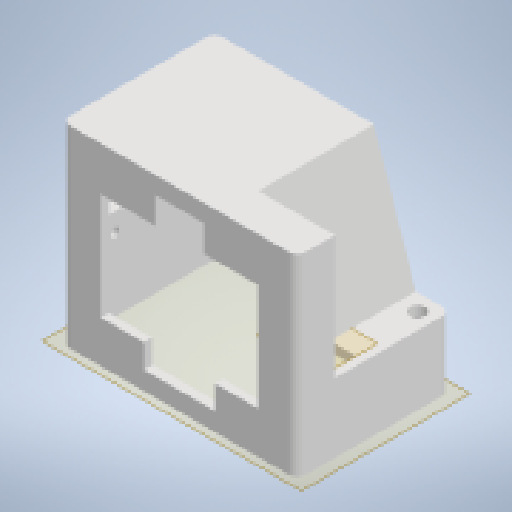
# Autodesk Inventor part: Gehaeuse_oben
Saved by Autodesk Inventor 2024 (Build 280153000, 153)
## iProperties
Created: 2025-04-09
Part Number: Gehaeuse_oben
Material: Generisch
Document SubType Name: Modeling
Designer: erikt
Density: 1 g/cm^3
Appearance: Vorgabe
Author: erikt
Autodesk Inventor part; units mm, degrees
ref_plane "YZ Plane" through (0, 0, 0) normal (1, 0, 0) x (0, 1, 0)
ref_plane "XZ Plane" through (0, 0, 0) normal (0, 1, 0) x (-1, 0, 0)
ref_plane "XY Plane" through (0, 0, 0) normal (0, 0, 1) x (1, 0, 0)
ref_plane "Arbeitsebene1" through (0, 0, 0) normal (0, 0, 1) x (1, 0, 0)
sketch "Skizze1" plane through (0, 0, 0) normal (0, 0, 1) x (1, 0, 0)
  arc A0 (-23.82, 16.765) -> (-25.82, 14.765) centre (-23.82, 14.765) ccw projected
  line L0 (-25.82, -14.765) -> (-25.82, 14.765) projected
  arc A1 (-25.82, -14.765) -> (-23.82, -16.765) centre (-23.82, -14.765) ccw projected
  line L1 (23.82, -16.765) -> (-23.82, -16.765) projected
  arc A2 (23.82, -16.765) -> (25.82, -14.765) centre (23.82, -14.765) ccw projected
  line L2 (25.82, 14.765) -> (25.82, -14.765) projected
  arc A3 (25.82, 14.765) -> (23.82, 16.765) centre (23.82, 14.765) ccw projected
  line L3 (-23.82, 16.765) -> (23.82, 16.765) projected
  arc A4 (23.82, -15.765) -> (24.82, -14.765) centre (23.82, -14.765) ccw projected
  line L4 (-23.82, -15.765) -> (23.82, -15.765) projected
  arc A5 (-24.82, -14.765) -> (-23.82, -15.765) centre (-23.82, -14.765) ccw projected
  line L5 (-24.82, 14.765) -> (-24.82, -14.765) projected
  arc A6 (-23.82, 15.765) -> (-24.82, 14.765) centre (-23.82, 14.765) ccw projected
  line L6 (23.82, 15.765) -> (-23.82, 15.765) projected
  arc A7 (24.82, 14.765) -> (23.82, 15.765) centre (23.82, 14.765) ccw projected
  line L7 (24.82, -14.765) -> (24.82, 14.765) projected
  arc A8 (-23.82, 15.965) -> (-25.02, 14.765) centre (-23.82, 14.765) ccw
  line L8 (-25.02, 14.765) -> (-25.02, -14.765)
  arc A9 (-25.02, -14.765) -> (-23.82, -15.965) centre (-23.82, -14.765) ccw
  line L9 (-23.82, -15.965) -> (23.82, -15.965)
  arc A10 (23.82, -15.965) -> (25.02, -14.765) centre (23.82, -14.765) ccw
  line L10 (25.02, -14.765) -> (25.02, 14.765)
  arc A11 (25.02, 14.765) -> (23.82, 15.965) centre (23.82, 14.765) ccw
  line L11 (23.82, 15.965) -> (-23.82, 15.965)
  point P0 (0, 0)
  dimension "d0" = 0.2
  constraints: 8 end point, 8 point on circle, 4 centre point, 7 other
  measures "d0" distance between parallel lines of L6 L11
extrude "Extrusion1" add sketch "Skizze1" along normal blind 2.2 contours L3 A3 L2 A2 L1 A1 L0 A0
sketch "Skizze2" plane through (0, 0, 2.2) normal (0, 0, 1) x (1, 0, 0)
  line L0 (23.82, 16.765) -> (-23.82, 16.765) projected
  line L1 (23.82, 14.765) -> (-23.82, 14.765) projected
  arc A0 (-24.82, -14.765) -> (-23.82, -15.765) centre (-23.82, -14.765) ccw projected
  line L2 (-23.82, -15.765) -> (23.82, -15.765) projected
  arc A1 (23.82, -15.765) -> (24.82, -14.765) centre (23.82, -14.765) ccw projected
  line L3 (24.82, -14.765) -> (24.82, 14.765) projected
  arc A2 (24.82, 14.765) -> (23.82, 15.765) centre (23.82, 14.765) ccw projected
  line L4 (23.82, 15.765) -> (-23.82, 15.765) projected
  arc A3 (-23.82, 15.765) -> (-24.82, 14.765) centre (-23.82, 14.765) ccw projected
  line L5 (-24.82, 14.765) -> (-24.82, -14.765) projected
  line L6 (-23.82, 14.765) -> (-23.82, -14.765) projected
  line L7 (23.82, 14.765) -> (-23.82, 14.765) projected
  line L8 (23.82, -14.765) -> (23.82, 14.765) projected
  line L9 (-23.82, -14.765) -> (23.82, -14.765) projected
  line L10 (23.82, 16.765) -> (-23.82, 16.765) projected
  arc A4 (-23.82, 16.765) -> (-25.82, 14.765) centre (-23.82, 14.765) ccw projected
  line L11 (-25.82, 14.765) -> (-25.82, -14.765) projected
  arc A5 (-25.82, -14.765) -> (-23.82, -16.765) centre (-23.82, -14.765) ccw projected
  line L12 (-23.82, -16.765) -> (23.82, -16.765) projected
  arc A6 (23.82, -16.765) -> (25.82, -14.765) centre (23.82, -14.765) ccw projected
  line L13 (25.82, -14.765) -> (25.82, 14.765) projected
  arc A7 (25.82, 14.765) -> (23.82, 16.765) centre (23.82, 14.765) ccw projected
  line L14 (-23.82, 15.965) -> (23.82, 15.965) projected
  arc A8 (25.02, 14.765) -> (23.82, 15.965) centre (23.82, 14.765) ccw projected
  line L15 (25.02, 14.765) -> (25.02, -14.765) projected
  arc A9 (23.82, -15.965) -> (25.02, -14.765) centre (23.82, -14.765) ccw projected
  line L16 (23.82, -15.965) -> (-23.82, -15.965) projected
  arc A10 (-25.02, -14.765) -> (-23.82, -15.965) centre (-23.82, -14.765) ccw projected
  line L17 (-25.02, -14.765) -> (-25.02, 14.765) projected
  arc A11 (-23.82, 15.965) -> (-25.02, 14.765) centre (-23.82, 14.765) ccw projected
  point P0 (0, 0)
extrude "Extrusion2" add sketch "Skizze2" along normal blind 38 contours A7 L13 A6 L12 A5 L11 A4 L0 | L5 A3 L4 A2 L3 A1 L2 A0 | L14 A8 L15 A9 L16 A10 L17 A11
sketch "Skizze3" plane through (-23.82, -16.765, 0) normal (0, -1, 0) x (1, 0, 0)
  line L0 (-2, 0) -> (-2, 40.2) projected
  line L1 (0, 40.2) -> (-2, 40.2) projected
  line L2 (0, 40.2) -> (47.64, 40.2) projected
  line L3 (49.64, 0) -> (49.64, 40.2) projected
  line L4 (49.64, 40.2) -> (47.64, 40.2) projected
  line L5 (49.64, 0) -> (47.64, 0) projected
  line L6 (0, 0) -> (47.64, 0) projected
  line L7 (-2, 0) -> (0, 0) projected
  line L8 (5.82, 38.2) -> (41.82, 38.2)
  line L9 (41.82, 38.2) -> (41.82, 4.2)
  line L10 (41.82, 4.2) -> (5.82, 4.2)
  line L11 (5.82, 4.2) -> (5.82, 38.2)
  point P0 (23.82, 0)
  dimension "d5" = 36
  dimension "d6" = 34
  dimension "d7" = 2
  dimension "d8" = 7.82
  dimension "d9" = 7.82
  constraints: 8 end point, 2 parallel, 1 horizontal, 1 perpendicular
  measures "d5" distance of L9.end L10.end
  measures "d6" distance of L8.end L9.end
  measures "d7" distance between parallel lines of L2 L8
  measures "d8" distance between parallel lines of L11 L0
  measures "d9" distance between parallel lines of L3 L9
extrude "Extrusion3" cut sketch "Skizze3" against normal up to surface (2 mm away) contours L8 L9 L10 L11
sketch "Skizze4" plane through (-23.82, -16.765, 0) normal (0, -1, 0) x (1, 0, 0)
  line L0 (5.82, 4.2) -> (5.82, 38.2) projected
  line L1 (5.82, 4.2) -> (5.82, 38.2) projected
  line L2 (5.82, 38.2) -> (41.82, 38.2) projected
  line L3 (41.82, 38.2) -> (41.82, 4.2) projected
  line L4 (41.82, 4.2) -> (5.82, 4.2) projected
  line L5 (0, 0) -> (47.64, 0) projected
  line L6 (47.64, 0) -> (47.64, 40.2) projected
  line L7 (0, 40.2) -> (47.64, 40.2) projected
  line L8 (0, 0) -> (0, 40.2) projected
  line L9 (42.02, 38.4) -> (5.62, 38.4)
  line L10 (5.62, 38.4) -> (5.62, 4)
  line L11 (5.62, 4) -> (42.02, 4)
  line L12 (42.02, 4) -> (42.02, 38.4)
  point P0 (23.82, 0)
  dimension "d12" = 0.2
  constraints: 8 end point, 3 other
  measures "d12" distance between parallel lines of L2 L9
extrude "Extrusion4" cut sketch "Skizze4" against normal up to surface (2 mm away) contours L12 L11 L10 L9
sketch "Skizze5" plane through (-23.82, -16.765, 0) normal (0, -1, 0) x (1, 0, 0)
  line L0 (5.62, 38.4) -> (42.02, 38.4) projected
  line L1 (42.02, 38.4) -> (42.02, 4) projected
  line L2 (42.02, 4) -> (5.62, 4) projected
  line L3 (5.62, 4) -> (5.62, 38.4) projected
  line L4 (0, 0) -> (47.64, 0) projected
  line L5 (47.64, 0) -> (47.64, 40.2) projected
  line L6 (0, 40.2) -> (47.64, 40.2) projected
  line L7 (0, 0) -> (0, 40.2) projected
  line L8 (31.32, 4.2) -> (31.32, 9.2) projected
  line L9 (31.32, 4.2) -> (41.82, 4.2) projected
  line L10 (41.82, 4.2) -> (41.82, 38.2) projected
  line L11 (41.82, 38.2) -> (5.82, 38.2) projected
  line L12 (5.82, 38.2) -> (5.82, 4.2) projected
  line L13 (5.82, 4.2) -> (16.32, 4.2) projected
  line L14 (16.32, 9.2) -> (16.32, 4.2) projected
  line L15 (31.32, 9.2) -> (16.32, 9.2) projected
  line L16 (40.82, 32.4) -> (6.82, 32.4) projected
  line L17 (40.82, 9.4) -> (40.82, 32.4) projected
  line L18 (6.82, 9.4) -> (40.82, 9.4) projected
  line L19 (6.82, 32.4) -> (6.82, 9.4) projected
  circle A0 centre (39.2325, 35.4875) radius 2.0875 projected
  circle A1 centre (8.4075, 35.4875) radius 2.0875 projected
  circle A2 centre (8.4075, 6.9125) radius 2.0875 projected
  circle A3 centre (39.2325, 6.9125) radius 2.0875 projected
  line L20 (28.63, 35.95) -> (26.63, 35.95) projected
  line L21 (26.63, 35.95) -> (26.63, 37.95) projected
  line L22 (26.63, 37.95) -> (28.63, 37.95) projected
  line L23 (28.63, 37.95) -> (28.63, 35.95) projected
  line L24 (26.09, 35.95) -> (24.09, 35.95) projected
  line L25 (24.09, 35.95) -> (24.09, 37.95) projected
  line L26 (24.09, 37.95) -> (26.09, 37.95) projected
  line L27 (26.09, 37.95) -> (26.09, 35.95) projected
  line L28 (21.55, 35.95) -> (21.55, 37.95) projected
  line L29 (21.55, 37.95) -> (23.55, 37.95) projected
  line L30 (23.55, 37.95) -> (23.55, 35.95) projected
  line L31 (23.55, 35.95) -> (21.55, 35.95) projected
  line L32 (19.01, 37.95) -> (21.01, 37.95) projected
  line L33 (21.01, 37.95) -> (21.01, 35.95) projected
  line L34 (21.01, 35.95) -> (19.01, 35.95) projected
  line L35 (19.01, 35.95) -> (19.01, 37.95) projected
  line L36 (6.62, 32.6) -> (41.02, 32.6)
  line L37 (41.02, 32.6) -> (41.02, 9.2)
  line L38 (41.02, 9.2) -> (6.62, 9.2)
  line L39 (6.62, 9.2) -> (6.62, 32.6)
  line L40 (19.01, 35.95) -> (28.63, 35.95)
  line L41 (28.63, 35.95) -> (28.63, 37.95)
  line L42 (28.63, 37.95) -> (19.01, 37.95)
  line L43 (19.01, 37.95) -> (19.01, 35.95)
  line L44 (29.13, 35.45) -> (18.51, 35.45)
  line L45 (18.51, 35.45) -> (18.51, 38.45)
  line L46 (18.51, 38.45) -> (29.13, 38.45)
  line L47 (29.13, 38.45) -> (29.13, 35.45)
  line L48 (16.02, 4.5) -> (6.12, 4.5)
  line L49 (6.12, 4.5) -> (6.12, 37.9)
  line L50 (6.12, 37.9) -> (41.52, 37.9)
  line L51 (41.52, 37.9) -> (41.52, 4.5)
  line L52 (41.52, 4.5) -> (31.62, 4.5)
  line L53 (31.62, 4.5) -> (31.62, 9.5)
  line L54 (31.62, 9.5) -> (16.02, 9.5)
  line L55 (16.02, 9.5) -> (16.02, 4.5)
  line L56 (16.02, 4.5) -> (16.02, 4)
  line L57 (31.62, 4.5) -> (31.62, 4)
  point P0 (23.82, 0)
  point P1 (31.62, 9.2)
  point P2 (29.13, 38.4)
  point P3 (18.51, 38.4)
  point P4 (16.02, 9.2)
  dimension "d15" = 0.2
  dimension "d16" = 0.5
  dimension "d17" = 0.3
  constraints: 44 end point, 4 parallel, 4 perpendicular, 2 point on line, 1 horizontal, 13 other
  measures "d15" distance between parallel lines of L16 L36
  measures "d16" distance between parallel lines of L40 L44
  measures "d17" distance between parallel lines of L14 L55
extrude "Extrusion5" add sketch "Skizze5" against normal blind 1.8 contours L0 L45 L11 L12 L13 L56 L2 L3 | L0 L1 L2 L57 L9 L10 L11 L47 | L45 L50 L49 L48 L56 L13 L12 L11 | L11 L10 L9 L57 L52 L51 L50 L47 | L45 L44 L47 L50 L51 L52 L53 L38 L37 L36 L39 L55 L48 L49 | A0 | A1 | A2 | A3
sketch "Skizze6" plane through (-23.82, 16.765, 0) normal (0, 1, 0) x (1, 0, 0)
  arc A0 (21.6432, -14.6) -> (20.1432, -13.1) centre (20.1432, -14.6) ccw projected
  line L0 (21.6432, -14.8) -> (21.6432, -14.6) projected
  arc A1 (20.1432, -16.3) -> (21.6432, -14.8) centre (20.1432, -14.8) ccw projected
  line L1 (14.1432, -16.3) -> (20.1432, -16.3) projected
  arc A2 (12.6432, -14.8) -> (14.1432, -16.3) centre (14.1432, -14.8) ccw projected
  line L2 (12.6432, -14.8) -> (12.6432, -14.6) projected
  arc A3 (14.1432, -13.1) -> (12.6432, -14.6) centre (14.1432, -14.6) ccw projected
  line L3 (20.1432, -13.1) -> (14.1432, -13.1) projected
  arc A4 (14.1432, -11.5) -> (11.0432, -14.6) centre (14.1432, -14.6) ccw
  line L4 (11.0432, -14.6) -> (11.0432, -14.8)
  arc A5 (11.0432, -14.8) -> (14.1432, -17.9) centre (14.1432, -14.8) ccw
  line L5 (14.1432, -17.9) -> (20.1432, -17.9)
  arc A6 (20.1432, -17.9) -> (23.2432, -14.8) centre (20.1432, -14.8) ccw
  line L6 (23.2432, -14.8) -> (23.2432, -14.6)
  arc A7 (23.2432, -14.6) -> (20.1432, -11.5) centre (20.1432, -14.6) ccw
  line L7 (20.1432, -11.5) -> (14.1432, -11.5)
  point P0 (23.82, 0)
  dimension "d20" = 1.6
  constraints: 8 end point, 8 point on circle, 4 centre point, 7 other
  measures "d20" distance between parallel lines of L3 L7
extrude "Extrusion6" cut sketch "Skizze6" against normal up to surface (2 mm away) contours L0 A1 L1 A2 L2 A3 L3 A0 | L7 A7 L6 A6 L5 A5 L4 A4
sketch "Skizze7" plane through (-23.82, -16.765, 0) normal (0, -1, 0) x (1, 0, 0)
  line L0 (31.62, 4) -> (16.02, 4) projected
  line L1 (16.02, 4) -> (16.02, 9.2) projected
  line L2 (16.02, 9.2) -> (6.62, 9.2) projected
  line L3 (6.62, 9.2) -> (6.62, 32.6) projected
  line L4 (6.62, 32.6) -> (41.02, 32.6) projected
  line L5 (41.02, 32.6) -> (41.02, 9.2) projected
  line L6 (41.02, 9.2) -> (31.62, 9.2) projected
  line L7 (31.62, 9.2) -> (31.62, 4) projected
  line L8 (29.13, 38.4) -> (29.13, 35.45) projected
  line L9 (29.13, 35.45) -> (18.51, 35.45) projected
  line L10 (18.51, 35.45) -> (18.51, 38.4) projected
  line L11 (18.51, 38.4) -> (29.13, 38.4) projected
  line L12 (0, 0) -> (47.64, 0) projected
  line L13 (47.64, 0) -> (47.64, 40.2) projected
  line L14 (0, 40.2) -> (47.64, 40.2) projected
  line L15 (0, 0) -> (0, 40.2) projected
  line L16 (18.51, 35.45) -> (29.13, 35.45)
  line L17 (29.13, 35.45) -> (29.13, 32.6)
  line L18 (29.13, 32.6) -> (18.51, 32.6)
  line L19 (18.51, 32.6) -> (18.51, 35.45)
  point P0 (23.82, 0)
  constraints: 8 end point, 2 parallel, 1 horizontal, 1 perpendicular, 1 point on line
extrude "Extrusion7" cut sketch "Skizze7" against normal up to surface (2 mm away) contours L4 L19 L9 L17
sketch "Skizze8" plane through (-23.82, -14.765, 2.2) normal (0, 1, 0) x (1, 0, 0)
  line L0 (41.82, -2) -> (41.82, -36) projected
  line L1 (41.82, -19) -> (47.64, -19)
  line L2 (47.64, 0) -> (47.64, -38) projected
  line L3 (45.98, -23) -> (43.48, -23)
  line L4 (43.48, -23) -> (43.48, -15)
  line L5 (43.48, -15) -> (45.98, -15)
  line L6 (45.98, -15) -> (45.98, -23)
  line L7 (45.98, -23) -> (43.48, -15) construction
  line L8 (43.48, -23) -> (45.98, -15) construction
  line L9 (5.82, -36) -> (5.82, -2) projected
  line L10 (5.62, -36.2) -> (5.62, -1.8) projected
  line L11 (5.62, -19) -> (0, -19)
  line L12 (0, 2.2) -> (0, -38) projected
  line L13 (4.06, -23) -> (1.56, -23)
  line L14 (1.56, -23) -> (1.56, -15)
  line L15 (1.56, -15) -> (4.06, -15)
  line L16 (4.06, -15) -> (4.06, -23)
  line L17 (4.06, -23) -> (1.56, -15) construction
  line L18 (1.56, -23) -> (4.06, -15) construction
  point P0 (23.82, 2.2)
  point P1 (44.73, -19)
  point P2 (2.81, -19)
  dimension "d25" = 2.5
  dimension "d26" = 8
  dimension "d27" = 2.5
  dimension "d28" = 8
  constraints: 28 end point, 9 midpoint, 4 parallel, 3 horizontal, 2 perpendicular, 1 point on line
  measures "d25" distance of L4.end L5.end
  measures "d26" distance of L3.end L4.end
  measures "d27" distance of L14.end L15.end
  measures "d28" distance of L13.end L14.end
extrude "Extrusion8" add sketch "Skizze8" along normal blind 5.5
sketch "Skizze9" plane through (19.66, -14.765, 17.2) normal (-1, 0, 0) x (0, 0, 1)
  line L0 (8, 0) -> (0, 0) projected
  line L1 (8, 0) -> (8, 5.5) projected
  line L2 (0, 5.5) -> (8, 5.5) projected
  line L3 (0, 0) -> (0, 5.5) projected
  line L4 (0, 0) -> (8, 0) projected
  line L5 (0, 0) -> (0, 5.5) projected
  line L6 (8, 5.5) -> (0, 5.5) projected
  line L7 (8, 0) -> (8, 5.5) projected
  line L8 (8, 5.5) -> (0, 5.5)
  line L9 (0, 5.5) -> (0, 2)
  line L10 (0, 2) -> (8, 2)
  line L11 (8, 2) -> (8, 5.5)
  line L12 (8, 2) -> (0, 5.5)
  line L13 (0, 5.5) -> (8, 5.5) projected
  line L14 (0, 2) -> (8, 5.5)
  circle A0 centre (4, 3.75) radius 1
  point P0 (-17.2, 14.765)
  dimension "d31" = 3.5
  dimension "d32" = 2
  constraints: 12 end point, 2 parallel, 1 centre point, 1 horizontal, 1 midpoint, 1 perpendicular, 1 point on line
  measures "d31" distance of L9.end L8.end
  measures "d32" diameter of A0
extrude "Extrusion9" cut sketch "Skizze9" against normal up to surface (2.5 mm away) contours A0 L14 L12 | L12 L14 A0 | A0 L12 L14 | L14 L12 A0
sketch "Skizze10" plane through (-19.76, -14.765, 25.2) normal (1, 0, 0) x (0, 0, -1)
  circle A0 centre (4, 3.75) radius 1 projected
  point P0 (25.2, 14.765)
extrude "Extrusion10" cut sketch "Skizze10" against normal up to surface (2.5 mm away)
sketch "Skizze11" plane through (-23.82, -9.265, 2.2) normal (0, 1, 0) x (1, 0, 0)
  line L0 (45.98, -23) -> (45.98, -15) projected
  line L1 (45.98, -15) -> (43.48, -15) projected
  line L2 (43.48, -15) -> (43.48, -23) projected
  line L3 (43.48, -23) -> (45.98, -23) projected
  line L4 (1.56, -15) -> (1.56, -23) projected
  line L5 (1.56, -23) -> (4.06, -23) projected
  line L6 (4.06, -23) -> (4.06, -15) projected
  line L7 (4.06, -15) -> (1.56, -15) projected
  point P0 (23.82, 2.2)
extrude "Extrusion11" add sketch "Skizze11" along normal blind 1
fillet "Rundung1" radius 2 4 edges at (-21.01, -8.265, 25.2) (20.91, -8.265, 25.2) (-21.01, -8.265, 17.2) (20.91, -8.265, 17.2)
ref_plane "Arbeitsebene2" through (9.72, -3.175, 15.1205) normal (0, 0, 1) x (0, -1, 0)
sketch "Skizze12" plane through (9.72, -3.175, 15.1205) normal (0, 0, 1) x (0, -1, 0)
  line L0 (5.35, 0) -> (5.35, 13.5) projected
  line L1 (11.59, 16.1) -> (-17.94, 16.1) projected
  line L2 (-17.94, 14.1) -> (11.59, 14.1) projected
  line L3 (5.35, 0) -> (-19.94, 0)
  line L4 (-19.94, 0) -> (-19.94, 16.1)
  line L5 (-19.94, 16.1) -> (5.35, 16.1)
  line L6 (5.35, 16.1) -> (5.35, 0)
  point P0 (-3.175, -9.72)
  point P1 (5.35, 16.1)
  point P2 (-17.94, 16.1)
  constraints: 8 end point, 2 parallel, 1 horizontal, 1 perpendicular
extrude "Extrusion12" cut sketch "Skizze12" along normal up to surface (25.0795 mm away)
sketch "Skizze13" plane through (-23.82, 16.765, 0) normal (0, 1, 0) x (1, 0, 0)
  line L0 (33.54, -15.1205) -> (47.64, -15.1205) projected
  line L1 (47.64, 0) -> (47.64, -15.1205) projected
  line L2 (47.64, 0) -> (0, 0) projected
  line L3 (0, 0) -> (0, -40.2) projected
  line L4 (33.54, -40.2) -> (0, -40.2) projected
  line L5 (33.54, -40.2) -> (33.54, -15.1205) projected
  arc A0 (23.2432, -14.6) -> (20.1432, -11.5) centre (20.1432, -14.6) ccw projected
  line L6 (23.2432, -14.6) -> (23.2432, -14.8) projected
  arc A1 (20.1432, -17.9) -> (23.2432, -14.8) centre (20.1432, -14.8) ccw projected
  line L7 (20.1432, -17.9) -> (14.1432, -17.9) projected
  arc A2 (11.0432, -14.8) -> (14.1432, -17.9) centre (14.1432, -14.8) ccw projected
  line L8 (11.0432, -14.8) -> (11.0432, -14.6) projected
  arc A3 (14.1432, -11.5) -> (11.0432, -14.6) centre (14.1432, -14.6) ccw projected
  line L9 (14.1432, -11.5) -> (20.1432, -11.5) projected
  line L10 (47.64, -15.1205) -> (49.64, -15.1205) projected
  line L11 (49.64, 0) -> (49.64, -15.1205) projected
  line L12 (49.64, 0) -> (47.64, 0) projected
  line L13 (47.64, 0) -> (47.64, -15.1205) projected
  line L14 (47.64, -40.2) -> (47.64, -15.1205) projected
  line L15 (49.64, -40.2) -> (47.64, -40.2) projected
  line L16 (49.64, -15.1205) -> (49.64, -40.2) projected
  line L17 (47.64, -15.1205) -> (49.64, -15.1205) projected
  line L18 (1.56, -17.2) -> (4.06, -17.2) projected
  line L19 (4.06, -17.2) -> (4.06, -25.2) projected
  line L20 (4.06, -25.2) -> (1.56, -25.2) projected
  line L21 (1.56, -25.2) -> (1.56, -17.2) projected
  line L22 (45.98, -25.2) -> (43.48, -25.2) projected
  line L23 (43.48, -25.2) -> (43.48, -17.2) projected
  line L24 (43.48, -17.2) -> (45.98, -17.2) projected
  line L25 (45.98, -17.2) -> (45.98, -25.2) projected
  line L26 (42.02, -38.4) -> (5.62, -38.4) projected
  line L27 (5.62, -38.4) -> (5.62, -4) projected
  line L28 (5.62, -4) -> (42.02, -4) projected
  line L29 (42.02, -4) -> (42.02, -38.4) projected
  line L30 (47.64, -2.2) -> (0, -2.2) projected
  line L31 (0, -2.2) -> (0, -40.2) projected
  line L32 (47.64, -40.2) -> (0, -40.2) projected
  line L33 (47.64, -2.2) -> (47.64, -40.2) projected
  line L34 (43.435, -12.1206) -> (42.94, -12.1206) projected
  line L35 (42.02, -15.1205) -> (33.54, -40.2)
  point P0 (23.82, 0)
  constraints: 2 end point, 2 point on line
extrude "Extrusion13" add sketch "Skizze13" against normal up to surface (2 mm away) contours L0 L35 L26 L5 | L26 L35 L5
sketch "Skizze15" plane through (0, 0, 40.2) normal (0, 0, 1) x (1, 0, 0)
  line L0 (25.82, -8.525) -> (23.82, -8.525) projected
  line L1 (23.82, -8.525) -> (23.82, -14.765) projected
  line L2 (23.82, -14.765) -> (-23.82, -14.765) projected
  line L3 (-23.82, -14.765) -> (-23.82, 14.765) projected
  line L4 (-23.82, 14.765) -> (9.72, 14.765) projected
  line L5 (9.72, 14.765) -> (9.72, 16.765) projected
  line L6 (9.72, 16.765) -> (-23.82, 16.765) projected
  arc A0 (-23.82, 16.765) -> (-25.82, 14.765) centre (-23.82, 14.765) ccw projected
  line L7 (-25.82, 14.765) -> (-25.82, -14.765) projected
  arc A1 (-25.82, -14.765) -> (-23.82, -16.765) centre (-23.82, -14.765) ccw projected
  line L8 (-23.82, -16.765) -> (23.82, -16.765) projected
  arc A2 (23.82, -16.765) -> (25.82, -14.765) centre (23.82, -14.765) ccw projected
  line L9 (25.82, -14.765) -> (25.82, -8.525) projected
  point P0 (0, 0)
extrude "Extrusion14" add sketch "Skizze15" along normal blind 2
sketch "Skizze17" plane through (-23.82, 14.765, 2.2) normal (0, -1, 0) x (1, 0, 0)
  line L0 (47.64, 12.9205) -> (42.02, 12.9205) projected
  line L1 (33.54, 38) -> (42.02, 12.9205) projected
  line L2 (33.54, 38) -> (33.54, 40) projected
  line L3 (0, 40) -> (33.54, 40) projected
  line L4 (0, 0) -> (0, 40) projected
  line L5 (0, 0) -> (47.64, 0) projected
  line L6 (47.64, 0) -> (47.64, 12.9205) projected
  arc A0 (20.1432, 9.3) -> (23.2432, 12.4) centre (20.1432, 12.4) ccw projected
  line L7 (20.1432, 9.3) -> (14.1432, 9.3) projected
  arc A1 (11.0432, 12.4) -> (14.1432, 9.3) centre (14.1432, 12.4) ccw projected
  line L8 (11.0432, 12.4) -> (11.0432, 12.6) projected
  arc A2 (14.1432, 15.7) -> (11.0432, 12.6) centre (14.1432, 12.6) ccw projected
  line L9 (14.1432, 15.7) -> (20.1432, 15.7) projected
  arc A3 (23.2432, 12.6) -> (20.1432, 15.7) centre (20.1432, 12.6) ccw projected
  line L10 (23.2432, 12.6) -> (23.2432, 12.4) projected
  line L11 (33.54, 38) -> (32.8637, 40)
  line L12 (0, 40) -> (33.54, 40) projected
  point P0 (23.82, -2.2)
  constraints: 2 end point, 1 point on line
extrude "Extrusion15" cut sketch "Skizze17" against normal blind 2 contours L11 L3 L2
sketch "Skizze18" plane through (-23.82, 14.765, 2.2) normal (0, -1, 0) x (1, 0, 0)
  arc A0 (20.1432, 9.3) -> (23.2432, 12.4) centre (20.1432, 12.4) ccw projected
  line L0 (20.1432, 9.3) -> (14.1432, 9.3) projected
  arc A1 (11.0432, 12.4) -> (14.1432, 9.3) centre (14.1432, 12.4) ccw projected
  line L1 (11.0432, 12.4) -> (11.0432, 12.6) projected
  arc A2 (14.1432, 15.7) -> (11.0432, 12.6) centre (14.1432, 12.6) ccw projected
  line L2 (14.1432, 15.7) -> (20.1432, 15.7) projected
  arc A3 (23.2432, 12.6) -> (20.1432, 15.7) centre (20.1432, 12.6) ccw projected
  line L3 (23.2432, 12.6) -> (23.2432, 12.4) projected
  line L4 (42.02, 12.9205) -> (32.8637, 40) projected
  line L5 (0, 40) -> (32.8637, 40) projected
  line L6 (0, 0) -> (0, 40) projected
  line L7 (0, 0) -> (47.64, 0) projected
  line L8 (47.64, 0) -> (47.64, 12.9205) projected
  line L9 (47.64, 12.9205) -> (42.02, 12.9205) projected
  line L10 (31.4288, 38) -> (40.585, 10.9205)
  line L11 (40.585, 10.9205) -> (45.64, 10.9205)
  line L12 (45.64, 10.9205) -> (45.64, 2)
  line L13 (45.64, 2) -> (2, 2)
  line L14 (2, 2) -> (2, 38)
  line L15 (2, 38) -> (31.4288, 38)
  line L16 (45.64, 10.9205) -> (47.64, 10.9205)
  line L17 (2, 38) -> (0, 38)
  point P0 (23.82, -2.2)
  dimension "d51" = 2
  constraints: 16 end point, 2 perpendicular, 2 point on line, 5 other
  measures "d51" distance between parallel lines of L5 L15
extrude "Extrusion16" add sketch "Skizze18" along normal up to surface (23.29 mm away) contours L9 L8 L16 L11 L10 L15 L17 L6 L5 L4
sketch "Skizze19" plane through (9.72, -3.175, 15.1205) normal (0, 0, 1) x (1, 0, 0)
  line L0 (16.1, -5.35) -> (14.1, -5.35) projected
  line L1 (14.1, -5.35) -> (16.1, -5.35) projected
  line L2 (8.48, 19.94) -> (8.48, -5.35) projected
  line L3 (14.1, -5.35) -> (8.48, -5.35)
  line L4 (8.48, -5.35) -> (8.48, 1.15)
  line L5 (8.48, 1.15) -> (14.1, 1.15)
  line L6 (14.1, 1.15) -> (14.1, -5.35)
  point P0 (-9.72, 3.175)
  point P1 (8.48, -5.35)
  dimension "d54" = 6.5
  constraints: 8 end point, 2 parallel, 1 horizontal, 1 perpendicular, 1 point on line
  measures "d54" distance of L3.end L4.end
extrude "Extrusion17" cut sketch "Skizze19" against normal blind 2
sketch "Skizze20" plane through (-23.82, -14.765, 2.2) normal (1, 0, 0) x (0, 0, -1)
  line L0 (-40, 0) -> (-40, 6.24) projected
  line L1 (-40, 0) -> (-38, 0)
  line L2 (-38, 0) -> (-38, 6.24)
  line L3 (-38, 6.24) -> (-40, 6.24)
  line L4 (-40, 6.24) -> (-40, 0)
  point P0 (2.2, 14.765)
  dimension "d57" = 2
  constraints: 8 end point, 2 parallel, 1 horizontal, 1 perpendicular
  measures "d57" distance of L3.end L2.end
extrude "Extrusion18" add sketch "Skizze20" along normal up to surface (47.64 mm away)
sketch "Skizze21" plane through (23.82, -14.765, 2.2) normal (-1, 0, 0) x (0, 0, 1)
  point P0 (-2.2, 14.765)
sketch "Skizze22" plane through (7.6088, -8.525, 40.2) normal (0, -1, 0) x (1, 0, 0)
  line L0 (2.1112, 0) -> (0, 0) projected
  line L1 (9.1563, -27.0795) -> (0, 0) projected
  line L2 (10.5912, -27.0795) -> (9.1563, -27.0795) projected
  line L3 (10.5912, -27.0795) -> (10.5912, -25.0795) projected
  line L4 (2.1112, 0) -> (10.5912, -25.0795) projected
  line L5 (2.1112, 0) -> (16.2112, 0) projected
  line L6 (16.2112, 0) -> (16.2112, -25.0795) projected
  line L7 (16.2112, -27.0795) -> (10.5912, -27.0795) projected
  line L8 (16.2112, 0) -> (16.2112, -25.0795) projected
  line L9 (16.2112, -25.0795) -> (16.2112, -27.0795) projected
  line L10 (16.2112, -38) -> (16.2112, -27.0795) projected
  line L11 (16.2112, -38) -> (16.2112, 0) projected
  point P0 (-7.6088, -40.2)
  point P1 (16.2112, -25.0795)
extrude "Extrusion19" add sketch "Skizze22" along normal blind 1
sketch "Skizze23" plane through (9.72, -3.175, 15.1205) normal (0, 0, 1) x (1, 0, 0)
  arc A0 (12.45, 17.94) -> (14.1, 16.29) centre (12.45, 16.29) ccw projected
  circle A1 centre (12.45, 16.29) radius 1.65
  point P0 (-9.72, 3.175)
  constraints: 1 centre point, 1 coincident, 1 concentric
extrude "Extrusion20" cut sketch "Skizze23" against normal blind 10
equation "\"d8\" = d9"
